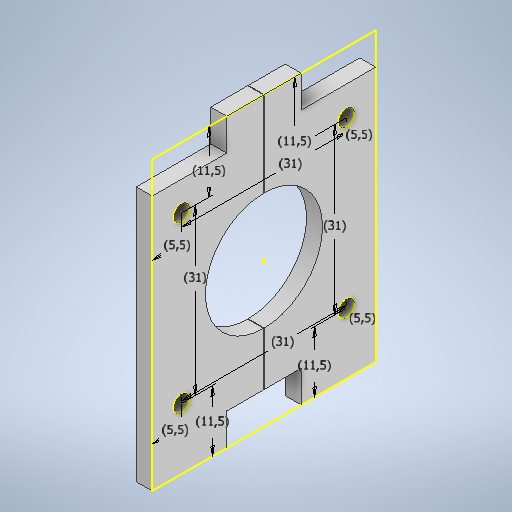
# Autodesk Inventor part: suporte do motor
Saved by Autodesk Inventor 2025.2 (Build 292293000, 293)
## iProperties
Created: 2025-05-20
Part Number: suporte do motor
Material: Genérico
Document SubType Name: Modeling
Designer: erick
Density: 1 g/cm^3
Appearance: Padrão
Author: erick
Autodesk Inventor part; units mm, degrees
ref_plane "YZ Plane" through (0, 0, 0) normal (1, 0, 0) x (0, 1, 0)
ref_plane "XZ Plane" through (0, 0, 0) normal (0, 1, 0) x (-1, 0, 0)
ref_plane "XY Plane" through (0, 0, 0) normal (0, 0, 1) x (1, 0, 0)
sketch "Esboço1" plane through (0, 0, 0) normal (1, 0, 0) x (0, 1, 0)
  line L0 (-27, 21) -> (27, 21)
  line L1 (27, 21) -> (27, -21)
  line L2 (27, -21) -> (-27, -21)
  line L3 (-27, -21) -> (-27, 21)
  line L4 (-27, 21) -> (27, -21) construction
  line L5 (27, 21) -> (-27, -21) construction
  point P0 (0, 0)
  dimension "d0" = 42
  dimension "d1" = 54
  constraints: 12 end point, 2 midpoint, 2 parallel, 1 horizontal, 1 perpendicular
  measures "d0" distance of L0.end L1.end
  measures "d1" distance of L1.end L2.end
extrude "Extrusão1" add sketch "Esboço1" along normal mid plane 3
sketch "Esboço2" plane through (1.5, 0, 0) normal (1, 0, 0) x (0, 0, -1)
  circle A0 centre (0, 0) radius 11
  dimension "d4" = 22
  constraints: 1 centre point, 1 coincident
  measures "d4" diameter of A0
extrude "Extrusão2" cut sketch "Esboço2" against normal through all
sketch "Esboço3" plane through (1.5, 0, 0) normal (1, 0, 0) x (0, 0, -1)
  circle A0 centre (-15.5, 15.5) radius 1.5
  line L0 (-21, 27) -> (-21, -27) projected
  line L1 (21, 27) -> (-21, 27) projected
  point P0 (0, 0)
  dimension "d7" = 5.5
  dimension "d8" = 3
  dimension "d9" = 11.5
  constraints: 1 centre point
  measures "d7" distance from line of L0 A0.centre
  measures "d8" diameter of A0
  measures "d9" distance from line of L1 A0.centre
extrude "Extrusão3" cut sketch "Esboço3" against normal through all
pattern_linear "Padrão retangular1" count 2 spacing 31 along (0, 0, -1) count 2 spacing 31 along (0, -1, 0) of "Extrusão3"
sketch "Esboço4" plane through (1.5, 0, 0) normal (1, 0, 0) x (0, 0, -1)
  line L0 (21, -27) -> (21, 27) projected
  circle A0 centre (15.5, 15.5) radius 1.5 projected
  line L1 (-21, 27) -> (-21, -27) projected
  circle A1 centre (-15.5, 15.5) radius 1.5 projected
  circle A2 centre (15.5, -15.5) radius 1.5 projected
  circle A3 centre (-15.5, -15.5) radius 1.5 projected
  line L2 (21, 27) -> (-21, 27) projected
  line L3 (-21, -27) -> (21, -27) projected
  point P0 (0, 0)
  dimension "d18" = 5.5
  dimension "d19" = 5.5
  dimension "d20" = 5.5
  dimension "d21" = 5.5
  dimension "d22" = 11.5
  dimension "d23" = 11.5
  dimension "d24" = 11.5
  dimension "d25" = 11.5
  dimension "d26" = 31
  dimension "d27" = 31
  dimension "d28" = 31
  dimension "d29" = 31
  measures "d18" distance from line of L0 A0.centre
  measures "d19" distance from line of L1 A1.centre
  measures "d20" distance from line of L0 A2.centre
  measures "d21" distance from line of L1 A3.centre
  measures "d22" distance from line of A1.centre L2
  measures "d23" distance from line of A0.centre L2
  measures "d24" distance from line of L3 A2.centre
  measures "d25" distance from line of L3 A3.centre
  measures "d26" distance of A0.centre A2.centre
  measures "d27" distance of A1.centre A3.centre
  measures "d28" distance of A0.centre A1.centre
  measures "d29" distance of A2.centre A3.centre
sketch "Esboço5" plane through (1.5, 0, 0) normal (1, 0, 0) x (0, 0, -1)
  line L0 (21, 27) -> (-21, 27) projected
  line L1 (-21, 27) -> (-7, 27)
  line L2 (-7, 27) -> (-7, 21)
  line L3 (-7, 21) -> (-21, 21)
  line L4 (-21, 21) -> (-21, 27)
  line L5 (21, 27) -> (7, 27)
  line L6 (7, 27) -> (7, 21)
  line L7 (7, 21) -> (21, 21)
  line L8 (21, 21) -> (21, 27)
  line L9 (-7, -33) -> (7, -33)
  line L10 (7, -33) -> (7, -21)
  line L11 (7, -21) -> (-7, -21)
  line L12 (-7, -21) -> (-7, -33)
  line L13 (-21, -27) -> (21, -27) projected
  line L14 (-7, -33) -> (7, -21) construction
  line L15 (7, -33) -> (-7, -21) construction
  line L16 (-21, 27) -> (-21, -27) projected
  line L17 (21, -27) -> (21, 27) projected
  point P0 (0, 0)
  point P1 (0, -27)
  point P2 (-7, -27)
  point P3 (7, -27)
  point P4 (7, 27)
  point P5 (-7, 27)
  dimension "d30" = 14
  dimension "d31" = 14
  dimension "d32" = 6
  dimension "d33" = 6
  dimension "d34" = 14
  dimension "d35" = 14
  dimension "d36" = 12
  dimension "d37" = 14
  dimension "d38" = 14
  dimension "d39" = 6
  constraints: 28 end point, 6 parallel, 3 horizontal, 3 midpoint, 3 perpendicular
  measures "d30" distance of L2.end L3.end
  measures "d31" distance of L6.end L7.end
  measures "d32" distance of L5.end L6.end
  measures "d33" distance of L1.end L2.end
  measures "d34" distance between parallel lines of L6 L2
  measures "d35" distance of L10.end L11.end
  measures "d36" distance of L9.end L10.end
  measures "d37" distance between parallel lines of L12 L16
  measures "d38" distance between parallel lines of L17 L10
  measures "d39" distance between parallel lines of L13 L11
extrude "Extrusão4" cut sketch "Esboço5" against normal through all contours L8 L7 L6 L0 | L2 L3 L4 L0 | L13 L12 L11 L10
sketch "Esboço6" plane through (1.5, 0, 0) normal (1, 0, 0) x (0, 0, -1)
  line L0 (-0.05, -30) -> (0.05, -30)
  line L1 (0.05, -30) -> (0.05, 30)
  line L2 (0.05, 30) -> (-0.05, 30)
  line L3 (-0.05, 30) -> (-0.05, -30)
  line L4 (-0.05, -30) -> (0.05, 30) construction
  line L5 (0.05, -30) -> (-0.05, 30) construction
  point P0 (0, 0)
  dimension "d44" = 60
  dimension "d45" = 0.1
  constraints: 12 end point, 2 midpoint, 2 parallel, 1 horizontal, 1 perpendicular
  measures "d44" distance of L0.end L1.end
  measures "d45" distance of L1.end L2.end
extrude "Extrusão5" cut sketch "Esboço6" against normal through all
